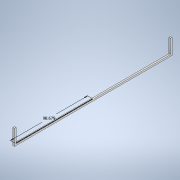
# Autodesk Inventor part: Part1
Saved by Autodesk Inventor 2020.2 (Build 242310000, 310)
## iProperties
Created: 2020-02-11
Part Number: Part1
Material: Generic
Document SubType Name: Modeling
Designer: ColinP
Density: 1 g/cm^3
Appearance: Default
Author: ColinP
Autodesk Inventor part; units mm, degrees
ref_plane "YZ Plane" through (0, 0, 0) normal (1, 0, 0) x (0, 1, 0)
ref_plane "XZ Plane" through (0, 0, 0) normal (0, 1, 0) x (-1, 0, 0)
ref_plane "XY Plane" through (0, 0, 0) normal (0, 0, 1) x (1, 0, 0)
sketch "Sketch1" plane through (0, 0, 0) normal (0, 1, 0) x (-1, 0, 0)
  line L0 (0, 0) -> (0, 98.679)
  line L1 (0, 0) -> (98.679, 0) construction
  line L2 (0, 98.679) -> (0, -98.679)
  line L3 (0, 98.679) -> (2, 98.679)
  line L4 (2, 98.679) -> (2, -98.679)
  line L5 (2, -98.679) -> (0, -98.679)
  line L6 (2, -98.679) -> (2, -100.679)
  line L7 (2, -100.679) -> (0, -100.679)
  line L8 (0, -100.679) -> (0, -98.679)
  line L9 (2, 98.679) -> (2, 100.679)
  line L10 (2, 100.679) -> (0, 100.679)
  line L11 (0, 100.679) -> (0, 98.679)
  dimension "d0" = 98.679
  dimension "d1" = 90
  dimension "d2" = 197.358
  dimension "d3" = 2
  dimension "d4" = 2
  dimension "d5" = 2
  constraints: 24 end point, 7 perpendicular, 4 point on line, 2 horizontal, 1 vertical
  measures "d0" distance of L0.start L0.end
  measures "d1" angle of L1 L0
  measures "d2" distance of L0.end L2.end
  measures "d3" distance of L0.end L3.end
  measures "d4" distance of L4.end L6.end
  measures "d5" distance of L3.end L9.end
extrude "Extrusion1" add sketch "Sketch1" along normal blind 2 contours L0 L3 L4 L5 L2
extrude "Extrusion2" add sketch "Sketch1" along normal blind 20 contours L11 L10 L9 L3 | L5 L6 L7 L8
sketch "Sketch2" plane through (0, 2, 0) normal (0, 1, 0) x (1, 0, 0)
  line L0 (-2, -98.679) -> (0, -98.679) projected
  line L1 (-1, -98.679) -> (-1, 0)
  point P0 (0, 0)
  dimension "d10" = 98.679
  constraints: 2 end point, 1 midpoint, 1 vertical
  measures "d10" distance of L1.start L1.end
body "Solid1"
